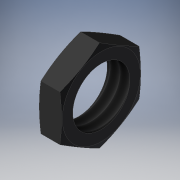
# Autodesk Inventor part: MN12P1(MNF12P1)
Saved by Autodesk Inventor 2019 (Build 230136000, 136)
## iProperties
Created: 2023-10-05
Part Number: MN12P1(MNF12P1)
Material: Generic
Catalog Web Link: www.cadenas.de
Description: Nut-
Vendor: PISCO_JP
Document SubType Name: Modeling
Designer: psAdmin
Manufacturer: PISCO_JP
Mass: 0.35438 g
Surface Area: 4.8921 cm^2
Volume: 0.35438 cm^3
Density: 1 g/cm^3
Appearance: PSOLRGB-175-175-175
Category: PARTsolutions
Company: PISCO_JP
Title: MN12P1(MNF12P1)
Author: Cadenas PARTsolutions
PSOL_IDENT_0: {$CADENAS_DATA/23d-libs/pisco_jp/vacuum_pad_series_r2/holder_joint/parts/nut.prj},167 {VTYP=3D},{NB=
PSOL_IDENT_1: MN12P1(MNF12P1)},{LINA=MN12P1(MNF12P1)},{NN=Nut},{DATE=19.06.2020 05:20:20},{GEOMDATE=24.09.2019 08:
PSOL_IDENT_2: 01:00},{VERSION=},{LINEID=90},{WBVAR=},{WBNUMERIC=}  {NB=MN12P1(MNF12P1)},{LINA=MN12P1(MNF12P1)},{KT=
PSOL_IDENT_3: DUMMY},{PARTNR=MN12P1(MNF12P1)},{REF=VPA-M4-6J},{VER=8}
NB: MN12P1(MNF12P1)
NN: Nut
NBSYN: $PARTNR.
LINA: MN12P1(MNF12P1)
CATALOG: NIHON PISCO CO., LTD
PARTNR: MN12P1(MNF12P1)
REF: VPA-M4-6J
VER: 8
SUPPLIER: PISCO_JP
ARTICLENO: MN12P1(MNF12P1)
BOMINFO: MN12P1(MNF12P1)
CREATOR: CADENAS GmbH
Autodesk Inventor part; units mm, degrees
sketch "Sketch_1" plane through (0, 0, 0) normal (0, 0, 1) x (1, 0, 0)
  line L0 (4, 0) -> (0, 0)
  line L1 (0, 0) -> (0, 6.9)
  line L2 (0, 6.9) -> (0.3698, 8.28)
  line L3 (0.3698, 8.28) -> (3.6302, 8.28)
  line L4 (3.6302, 8.28) -> (4, 6.9)
  line L5 (4, 6.9) -> (4, 0)
  line L6 (4, 0) -> (0, 0)
  constraints: 14 end point
revolve "Revolution1" add sketch "Sketch_1" angle 360 about axis through (4, 0, 0) along (1, 0, 0)
sketch "Sketch2" plane through (0, 0, 0) normal (-1, 0, 0) x (0, 0, 1)
  point P0 (0, 0)
hole "Hole1" at (0, 0, 0) direction (1, 0, 0) diameter 10.106 depth 4 thread size "M12x1.75" class "6H" standard "ISO Metric profile"
sketch "Sketch_3" plane through (0, 0, 0) normal (1, 0, 0) x (0, 1, 0)
  line L0 (14, 14) -> (-14, 14)
  line L1 (-14, 14) -> (-14, -14)
  line L2 (-14, -14) -> (14, -14)
  line L3 (14, -14) -> (14, 14)
  line L4 (-4.0415, 7) -> (-8.0829, 0)
  line L5 (-8.0829, 0) -> (-4.0415, -7)
  line L6 (-4.0415, -7) -> (4.0415, -7)
  line L7 (4.0415, -7) -> (8.0829, 0)
  line L8 (8.0829, 0) -> (4.0415, 7)
  line L9 (4.0415, 7) -> (-4.0415, 7)
  constraints: 20 end point
extrude "Extrusion1" cut sketch "Sketch_3" along normal blind 4
ref_plane "IP_Holder_XY" through (0, 0, 0) normal (-1, 0, 0) x (0, 0, -1)
ref_plane "IP_Holder_YZ" through (0, 0, 0) normal (0, 0, -1) x (0, -1, 0)
ref_plane "IP_Holder_ZX" through (0, 0, 0) normal (0, -1, 0) x (-1, 0, 0)
body "Solid1"
